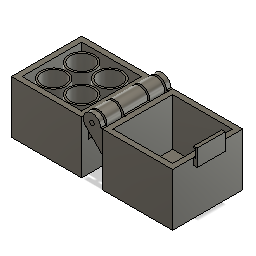
pudelko-hex (Autodesk Fusion 360 design; units mm, degrees)
Autodesk Fusion 360 part; units mm, degrees
note: some values were not read from the file. Chosen so that the rebuilt part matches the saved one: which bodies a step acts on; which face or edge a step refers to. Set by a fixed rule: which sketch regions a step uses.
sketch "Sketch1" plane through (0, 0, 0) normal (0, 1, 0) x (1, 0, 0)
  line L0 (-10, 10) -> (10, 10)
  line L1 (10, 10) -> (10, -10)
  line L2 (10, -10) -> (-10, -10)
  line L3 (-10, -10) -> (-10, 10)
  constraint horizontal L0
  constraint vertical L1
  constraint horizontal L2
  constraint vertical L3
extrude "Extrude1" add sketch "Sketch1" along normal blind 30 makes body 1
shell "Shell1" thickness 1.5 removed faces 0 bodies 1
ref_plane "WorkPlane1" through (0, 15, 0) normal (0, 1, 0) x (0, 0, 1)
split "Split1" by plane through (0, 15, 0) normal (0, 1, 0) bodies 1 makes body 2 at (-3.3333, 30, -3.3333)
sketch "Hinge" plane through (0, 0, 10) normal (0, 0, 1) x (1, 0, 0)
  line L0 (10, 15) -> (-10, 15)
  line L1 (-10, 15) -> (-10, 0)
  line L2 (-10, 0) -> (10, 0)
  line L3 (10, 0) -> (10, 15)
  line L4 (10, 15) -> (12.95, 15)
  circle A0 centre (12.95, 15) radius 2.45
  circle A1 centre (12.95, 15) radius 1.15
  circle A2 centre (12.95, 15) radius 0.65
  line L5 (10, 8.5852) -> (14.6824, 13.2676)
  line L6 (10, 15) -> (10, 30)
  line L7 (10, 21.4148) -> (14.6824, 16.7324)
  dimension "d5" = 2.95
  dimension "d6" = 1.3
  dimension "d7" = 0.5
  dimension "d8" = 1.3
  dimension "d9" = 45
  dimension "d11" = 45
  constraint coincident L0.start L3.end
  constraint perpendicular L3 L4
  constraint coincident L4.end A0.centre
  constraint concentric A0 A1
  constraint concentric A0 A2
  constraint coincident L3 L5.start
  constraint coincident A0 L5.end
  constraint tangent A0 L5
  constraint coincident L6 L7.start
  constraint coincident A0 L7.end
  constraint tangent A0 L7
  measures "d5" distance of L0.start L4.end
  measures "d6" diameter of A2
  measures "d7" distance of A1 A2
  measures "d8" distance of A0 A1
  measures "d9" angle of L3 L5
  measures "d11" angle of L6 L7
extrude "Extrude2" add sketch "Hinge" against normal up to surface (20 mm away) separate body contours L3 L4 A0 L5 | A0 makes body 3
extrude "Extrude3" add sketch "Hinge" against normal up to surface (20 mm away) separate body contours L4 A0 L6 L7 | A0 | A1 | A2 makes body 4
extrude "Extrude4" add sketch "Hinge" against normal up to surface (20 mm away) separate body contours A2 makes body 5
sketch "Sketch3" plane through (0, 15, 0) normal (0, 1, 0) x (-1, 0, 0)
  line L0 (10, -10) -> (10, 10)
  line L1 (10, 10) -> (-10, 10)
  line L2 (-10, 10) -> (-10, -10)
  line L3 (-10, -10) -> (10, -10)
  line L4 (8.5, 8.5) -> (8.5, -8.5)
  line L5 (8.5, -8.5) -> (-8.5, -8.5)
  line L6 (-8.5, -8.5) -> (-8.5, 8.5)
  line L7 (-8.5, 8.5) -> (8.5, 8.5)
  line L8 (-10, 10) -> (-15.5, 10)
  line L9 (-15.5, 10) -> (-15.5, 8.7)
  line L10 (-15.5, 8.7) -> (-10, 8.7)
  line L11 (-10, 8.7) -> (-10, 10)
  line L12 (-10, 8.7) -> (-15.5, 8.7)
  line L13 (-15.5, 8.7) -> (-15.5, 8.2)
  line L14 (-15.5, 8.2) -> (-10, 8.2)
  line L15 (-10, 8.2) -> (-10, 8.7)
  line L16 (-10, 0) -> (-16, 0) construction
  line L17 (-10, 0) -> (-10, 3.5) construction
  line L18 (-10, 3.5) -> (-15.5, 3.5)
  line L19 (-15.5, 3.5) -> (-15.5, 4)
  line L20 (-15.5, 4) -> (-10, 4)
  line L21 (-10, 4) -> (-10, 3.5)
  line L22 (-15.5, -10) -> (-15.5, -8.7)
  line L23 (-10, -4) -> (-10, -3.5)
  line L24 (-10, -8.7) -> (-10, -10)
  line L25 (-10, -3.5) -> (-15.5, -3.5)
  line L26 (-15.5, -3.5) -> (-15.5, -4)
  line L27 (-10, -8.2) -> (-10, -8.7)
  line L28 (-15.5, -4) -> (-10, -4)
  line L29 (-10, -10) -> (-15.5, -10)
  line L30 (-15.5, -8.7) -> (-15.5, -8.2)
  line L31 (-10, -8.7) -> (-15.5, -8.7)
  line L32 (-15.5, -8.2) -> (-10, -8.2)
  line L33 (-15.5, -8.7) -> (-10, -8.7)
  point P0 (-10, -10)
  dimension "d18" = 5.5
  dimension "d19" = 1.3
  dimension "d20" = 5.5
  dimension "d21" = 0.5
  dimension "d22" = 3.5
  dimension "d23" = 5.5
  dimension "d24" = 0.5
  constraint horizontal L8
  constraint vertical L9
  constraint horizontal L10
  constraint vertical L11
  constraint coincident L1.end L2.start
  constraint horizontal L12
  constraint vertical L13
  constraint horizontal L14
  constraint vertical L15
  constraint midpoint L2 L16.start
  constraint perpendicular L2 L16
  constraint perpendicular L16 L17
  constraint horizontal L18
  constraint vertical L19
  constraint horizontal L20
  constraint vertical L21
  constraint symmetric L1.end L16 P0
  constraint symmetric L8.end L16 L22.start
  constraint symmetric L9.end L16 L22.end
  constraint symmetric L10.end L16 L24.start
  constraint symmetric L13.end L16 L30.end
  constraint symmetric L14.end L16 L27.start
  constraint symmetric L16 L17.end L23.end
  constraint symmetric L16 L18.end L25.end
  constraint symmetric L16 L19.end L26.end
  constraint symmetric L16 L20.end L23.start
  measures "d18" distance of L1.end L8.end
  measures "d19" distance of L1.end L10.end
  measures "d20" distance of L10.end L9.end
  measures "d21" distance of L10.end L14.end
  measures "d22" distance of L16.start L17.end
  measures "d23" distance of L17.end L18.end
  measures "d24" distance of L17.end L20.end
extrude "Extrude5" cut sketch "Sketch3" along normal through all and the other way through all contours L2 L27 L30 L31 L32 L33 | L2 L10 L12 L13 L14 L15 | L2 L23 L25 L26 L28 | L2 L18 L19 L20 L21 bodies 3 4 makes body 10 at (10.5115, 14.7628, -5.4) makes body 11 at (11.7275, 17.7157, 10) makes body 12 at (10.5115, 14.7628, 6.8) makes body 13 at (11.7275, 17.7157, -8.7) makes body 6 at (14.7959, 16.6109, -5.4) makes body 7 at (10.7443, 12.562, 8.7) makes body 8 at (14.7959, 16.6109, 1.1667) makes body 9 at (10.7443, 12.562, -8.7)
delete_body "RemoveBody1" bodies 8
delete_body "RemoveBody2" bodies 10
delete_body "RemoveBody3" bodies 12
copy_body "Body->Comp1" bodies 2 removing the originals makes body 14 in component "Top Box"
copy_body "CutPasteBodies1" bodies 1 7 11 13 9 4 5 6 3 removing the originals makes body 15 makes body 16 makes body 17 makes body 18 makes body 19 makes body 20 makes body 21 makes body 22 makes body 23 in component "Bottom Box"
copy_body "CutPasteBodies1'" bodies 17 removing the originals makes body 24 in component "Top Box"
copy_body "CutPasteBodies2" bodies 18 removing the originals makes body 25 in component "Top Box"
copy_body "CutPasteBodies3" bodies 20 removing the originals makes body 26 in component "Top Box"
copy_body "CutPasteBodies4" bodies 21 removing the originals makes body 27 in component "Top Box"
sketch "Sketch4" plane through (0, 1.5, 0) normal (0, 1, 0) x (-1, 0, 0)
  line L0 (8.5, 8.5) -> (-8.5, 8.5)
  line L1 (-8.5, 8.5) -> (-8.5, -8.5)
  line L2 (-8.5, -8.5) -> (8.5, -8.5)
  line L3 (8.5, -8.5) -> (8.5, 8.5)
  circle A0 centre (4, 4) radius 3.2
  circle A1 centre (4, 4) radius 3.7
  line L4 (8.5, 0) -> (-8.5, 0) construction
  line L5 (0, 8.5) -> (0, -8.5) construction
  circle A2 centre (4, -4) radius 3.7
  circle A3 centre (4, -4) radius 3.2
  circle A4 centre (-4, 4) radius 3.2
  circle A5 centre (-4, 4) radius 3.7
  circle A6 centre (-4, -4) radius 3.7
  circle A7 centre (-4, -4) radius 3.2
  dimension "d32" = 6.4
  dimension "d33" = 7.4
  constraint midpoint L3 L4.start
  constraint midpoint L1 L4.end
  constraint midpoint L0 L5.start
  constraint midpoint L2 L5.end
  constraint symmetric A0 L4 A3
  constraint symmetric A1 L4 A2
  constraint symmetric A0 L5 A4
  constraint symmetric A1 L5 A5
  constraint symmetric L5 A2 A6
  constraint symmetric L5 A3 A7
  measures "d32" diameter of A0
  measures "d33" diameter of A1
extrude "Extrude1'" add sketch "Sketch4" along normal blind 13 contours A5 bodies 15 in component "Bottom Box"
extrude "Extrude2'" add sketch "Sketch4" along normal blind 13 contours A1 | A2 | A6 bodies 15 in component "Bottom Box"
sketch "Sketch5" plane through (-10, 0, 0) normal (-1, 0, 0) x (0, 0, 1)
  line L0 (10, 15) -> (-10, 15)
  line L1 (-10, 15) -> (-10, 0)
  line L2 (-10, 0) -> (10, 0)
  line L3 (10, 0) -> (10, 15)
  line L4 (-4, 11) -> (4, 11)
  line L5 (4, 11) -> (4, 7)
  line L6 (4, 7) -> (-4, 7)
  line L7 (-4, 7) -> (-4, 11)
  constraint horizontal L4
  constraint vertical L5
  constraint horizontal L6
  constraint vertical L7
extrude "Extrude6" add sketch "Sketch5" along normal blind 0.5 separate body contours L4 L5 L6 L7 makes body 28
copy_body "CutPasteBodies2'" bodies 28 removing the originals makes body 29 in component "Bottom Box"
fillet "Fillet1" radius 5 1 edges at (-10.5, 11, 0) on bodies 29 in component "Bottom Box"
move_face "OffsetFaces1" offset -1.85 1 faces at (-10.3333, 7, 1.3333) on bodies 29 in component "Bottom Box"
move_body "Move1" bodies 29 to x (1, 0, 0) y (0, 1, 0) z (0, 0, 1) at (0, 3.8, 0) in component "Bottom Box"
sketch "Sketch7" plane through (-10, 0, 0) normal (-1, 0, 0) x (0, 0, 1)
  line L0 (-10, 15) -> (10, 15)
  line L1 (10, 15) -> (10, 30)
  line L2 (10, 30) -> (-10, 30)
  line L3 (-10, 30) -> (-10, 15)
  line L4 (-4, 17) -> (4, 17)
  line L5 (4, 17) -> (4, 11)
  line L6 (4, 11) -> (-4, 11)
  line L7 (-4, 11) -> (-4, 17)
  constraint horizontal L4
  constraint vertical L5
  constraint horizontal L6
  constraint vertical L7
extrude "Extrude7" add sketch "Sketch7" along normal blind 0.8 separate body contours L0 L4 L5 L7 | L0 L5 L6 L7 makes body 30
copy_body "CutPasteBodies5" bodies 30 removing the originals makes body 31 in component "Top Box"
move_face "OffsetFaces1'" offset -1.2 1 faces at (-10.2667, 11, 1.3333) on bodies 31 in component "Top Box"
sketch "Sketch8" plane through (0, 0, 4) normal (0, 0, 1) x (1, 0, 0)
  line L0 (-10, 12.2) -> (-10, 17)
  line L1 (-10, 17) -> (-10.8, 17)
  line L2 (-10.8, 17) -> (-10.8, 12.2)
  line L3 (-10.8, 12.2) -> (-10, 12.2)
  line L4 (-10, 15) -> (-10.6, 15)
  line L5 (-10.6, 15) -> (-10.6, 12.6)
  line L6 (-10.6, 12.6) -> (-10, 12.6)
  line L7 (-10, 12.6) -> (-10, 15)
  dimension "d47" = 0.6
  dimension "d48" = 2.4
  constraint horizontal L4
  constraint vertical L5
  constraint horizontal L6
  constraint vertical L7
  constraint coincident L0 L4.start
  measures "d47" distance of L4.start L4.end
  measures "d48" distance of L4.start L6.end
extrude "Extrude1''" cut sketch "Sketch8" against normal blind 9 contours L0 L4 L5 L6 L7 bodies 31 in component "Top Box"
extrude "Extrude2''" add 1 faces at (-10.8, 13.8, 1.3333) along direction (-1, 0, 0) blind 0.2 on bodies 31 bodies 31 in component "Top Box"
delete_body "RemoveBody5" bodies 16 in component "Bottom Box"
delete_body "RemoveBody6" bodies 19 in component "Bottom Box"
component "Top Box" placed x (1, 0, 0) y (0, 1, 0) z (0, 0, 1) at (0, 0, 0)
component "Bottom Box" placed x (1, 0, 0) y (0, 1, 0) z (0, 0, 1) at (0, 0, 0)
named bodies: "Bottom", "Top", "Bottom Hinge", "Top Hinge", "Pin", "Bottom Hinge (1)", "Bottom Hinge (2)", "Bottom Hinge (3)", "Bottom Hinge (4)", "Top Hinge (1)", "Top Hinge (2)", "Top Hinge (3)", "Top Hinge (4)", "Hook", "Latch"
